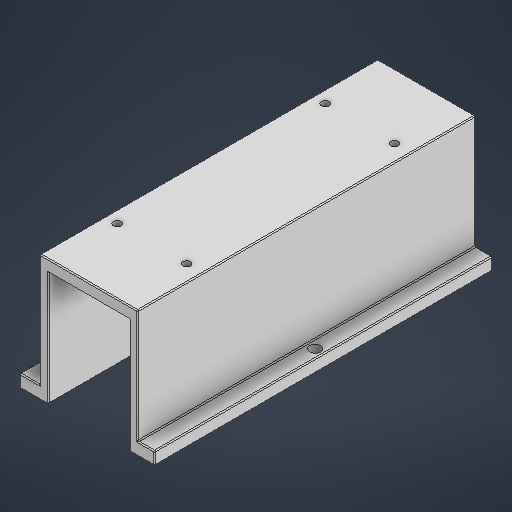
# Autodesk Inventor part: controllerHousing
Saved by Autodesk Inventor 2026 (Build 300175000, 175)
## iProperties
Created: 2025-04-15
Part Number: controllerHousing
Material: Generic
Document SubType Name: Modeling
Designer: Elizabeth
Density: 1 g/cm^3
Appearance: Default
Author: Elizabeth
Autodesk Inventor part; units mm, degrees
ref_plane "YZ Plane" through (0, 0, 0) normal (1, 0, 0) x (0, 1, 0)
ref_plane "XZ Plane" through (0, 0, 0) normal (0, 1, 0) x (-1, 0, 0)
ref_plane "XY Plane" through (0, 0, 0) normal (0, 0, 1) x (1, 0, 0)
sketch "Sketch1" plane through (0, 0, 0) normal (0, 1, 0) x (-1, 0, 0)
  line L0 (-40, 0) -> (-40, -100)
  line L1 (0, -100) -> (0, 0)
  line L2 (-35, 0) -> (-35, -100)
  line L3 (-6, -100) -> (-6, 0)
  circle A0 centre (-2.5, -50) radius 1.65
  circle A1 centre (-37.5, -50) radius 1.65
  line L4 (0, 0) -> (-8.5, 0)
  line L5 (-32.5, 0) -> (-40, 0)
  line L6 (-40, -100) -> (-32.5, -100)
  line L7 (-8.5, -100) -> (0, -100)
  line L8 (-8.5, 0) -> (-8.5, -100)
  line L9 (-32.5, -100) -> (-32.5, 0)
  dimension "d4" = 3.3
  dimension "d5" = 3.3
  dimension "d8" = 2.5
  dimension "d9" = 2.5
  constraints: 20 end point, 6 parallel, 4 point on line, 2 centre point, 2 horizontal, 2 perpendicular
  measures "d4" diameter of A0
  measures "d5" diameter of A1
  measures "d8" distance between parallel lines of L3 L8
  measures "d9" distance between parallel lines of L2 L9
extrude "Extrusion1" add sketch "Sketch1" along normal blind 3.5
sketch "Sketch2" plane through (0, 3.5, 0) normal (0, 1, 0) x (1, 0, 0)
  line L0 (8.5, 100) -> (0, 100) projected
  line L1 (8.5, 100) -> (6, 100)
  line L2 (6, 100) -> (6, 0)
  line L3 (6, 0) -> (8.5, 0)
  line L4 (8.5, 0) -> (8.5, 100)
  line L5 (32.5, 100) -> (32.5, 0) projected
  line L6 (32.5, 100) -> (35, 100)
  line L7 (35, 100) -> (35, 0)
  line L8 (35, 0) -> (32.5, 0)
  line L9 (32.5, 0) -> (32.5, 100)
  point P0 (0, 0)
  point P1 (32.5, 0)
  point P2 (6, 100)
  dimension "d10" = 2.5
  dimension "d11" = 100
  dimension "d12" = 2.5
  dimension "d13" = 100
  constraints: 16 end point, 4 parallel, 2 horizontal, 2 perpendicular
  measures "d10" distance of L3.end L2.end
  measures "d11" distance of L2.end L1.end
  measures "d12" distance of L7.end L8.end
  measures "d13" distance of L6.end L7.end
extrude "Extrusion2" add sketch "Sketch2" along normal blind 30
sketch "Sketch3" plane through (0, 33.5, 0) normal (0, 1, 0) x (1, 0, 0)
  line L0 (6, 100) -> (6, 0) projected
  line L1 (35, 100) -> (35, 0) projected
  line L2 (6, 0) -> (35, 0)
  line L3 (35, 0) -> (35, 100)
  line L4 (35, 100) -> (6, 100)
  line L5 (6, 100) -> (6, 0)
  point P0 (0, 0)
  point P1 (35, 0)
  point P2 (6, 100)
  constraints: 8 end point, 2 parallel, 1 horizontal, 1 perpendicular
extrude "Extrusion3" add sketch "Sketch3" along normal blind 3.5
sketch "Sketch4" plane through (0, 37, 0) normal (0, 1, 0) x (1, 0, 0)
  circle A0 centre (9.75, 80.75) radius 1.15
  circle A1 centre (30.25, 80.75) radius 1.15
  circle A2 centre (9.75, 19.25) radius 1.15
  circle A3 centre (30.25, 19.25) radius 1.15
  point P0 (0, 0)
  constraints: 4 centre point
extrude "Extrusion4" cut sketch "Sketch4" against normal blind 3.5
fillet "Fillet1" radius 0.3 24 edges at (6, 20.25, -100) (3, 3.5, -100) (20.5, 37, -100) (8.5, 16.75, -100) (20.5, 33.5, -100) (35, 20.25, -100) (32.5, 16.75, -100) (32.5, 16.75, 0) (35, 20.25, 0) (20.5, 37, 0) (20.5, 33.5, 0) (8.5, 16.75, 0) (6, 20.25, 0) (6, 37, -50) (35, 37, -50) (0, 3.5, -50) (40, 3.5, -50) (37.5, 3.5, 0) (3, 3.5, 0) (0, 1.75, 0) (40, 1.75, 0) (40, 1.75, -100) (37.5, 3.5, -100) (0, 1.75, -100)
fillet "Fillet2" radius 0.3 6 edges at (6.0879, 3.4121, -99.9121) (6.0879, 3.4121, -0.0879) (6, 3.5, -50) (34.9121, 3.4121, -0.0879) (34.9121, 3.4121, -99.9121) (35, 3.5, -50)
body "Solid1"
